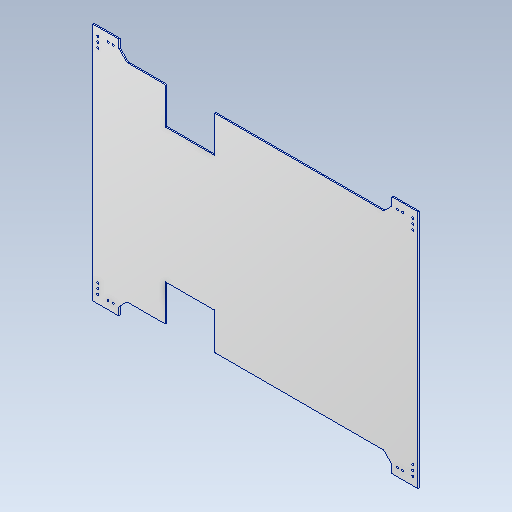
# Autodesk Inventor part: BELLYPAN
Saved by Autodesk Inventor 2020 (Build 240168000, 168)
## iProperties
Created: 2021-01-06
Part Number: BELLYPAN
Material: Aluminum 6061
Document SubType Name: Modeling
Designer: lucky
Density: 2.7 g/cm^3
Appearance: Aluminum - Flat
Mass: 3216.38 g
Surface Area: 8048.59 cm^2
Volume: 1191.25 cm^3
Author: lucky
Autodesk Inventor part; units mm, degrees
ref_plane "YZ Plane" through (0, 0, 0) normal (1, 0, 0) x (0, 1, 0)
ref_plane "XZ Plane" through (0, 0, 0) normal (0, 1, 0) x (-1, 0, 0)
ref_plane "XY Plane" through (0, 0, 0) normal (0, 0, 1) x (1, 0, 0)
sketch "Sketch1" plane through (0, 0, 0) normal (0, 0, 1) x (1, 0, 0)
  line L0 (775, 52) -> (25, 52) projected
  line L1 (0, 0) -> (0, 700) projected
  line L2 (0, 52) -> (800, 52)
  line L3 (800, 52) -> (800, 642)
  line L4 (800, 642) -> (0, 642)
  line L5 (0, 642) -> (0, 52)
  point P0 (0, 642)
  dimension "d0" = 800
  dimension "d1" = 590
  constraints: 8 end point, 2 parallel, 1 horizontal, 1 perpendicular, 1 point on line
  measures "d0" distance between parallel lines of L3 L1
  measures "d1" distance between parallel lines of L0 L4
extrude "Extrusion1" add sketch "Sketch1" along normal blind 3
sketch "Sketch2" plane through (0, 0, 3) normal (0, 0, 1) x (1, 0, 0)
  line L0 (25, 642) -> (775, 642) projected
  line L1 (671.5125, 642) -> (700.0875, 642) projected
  line L2 (800, 642) -> (0, 642) projected
  line L3 (735.75, 642) -> (64.25, 642)
  line L4 (64.25, 642) -> (64.25, 622)
  line L5 (84.25, 602) -> (715.75, 602)
  line L6 (735.75, 622) -> (735.75, 642)
  line L7 (800, 52) -> (800, 642) projected
  line L8 (0, 642) -> (0, 52) projected
  line L9 (0, 52) -> (800, 52) projected
  line L10 (735.75, 52) -> (64.25, 52)
  line L11 (64.25, 52) -> (64.25, 72)
  line L12 (84.25, 92) -> (715.75, 92)
  line L13 (735.75, 72) -> (735.75, 52)
  line L14 (25, 602) -> (775, 602) projected
  line L15 (270.7648, 597) -> (270.7648, 602) projected
  line L16 (178.8488, 568.7508) -> (178.8488, 563.7508) projected
  line L17 (178.2661, 125.2492) -> (178.2661, 130.2492) projected
  line L18 (299.9157, 125.2492) -> (299.9157, 130.2492) projected
  line L19 (300.4983, 568.7508) -> (300.4983, 563.7508) projected
  line L20 (298.8488, 602) -> (178.8488, 602)
  line L21 (178.8488, 602) -> (178.8488, 512)
  line L22 (178.8488, 512) -> (298.8488, 512)
  line L23 (298.8488, 512) -> (298.8488, 602)
  line L24 (800, 347) -> (0, 347) construction
  line L25 (178.8488, 92) -> (178.8488, 182)
  line L26 (178.8488, 182) -> (298.8488, 182)
  line L27 (298.8488, 182) -> (298.8488, 92)
  line L28 (64.25, 622) -> (84.25, 602)
  line L29 (735.75, 622) -> (715.75, 602)
  line L30 (84.25, 92) -> (64.25, 72)
  line L31 (715.75, 92) -> (735.75, 72)
  point P0 (0, 0)
  point P1 (64.25, 602)
  point P2 (735.75, 602)
  point P3 (64.25, 92)
  point P4 (735.75, 92)
  point P5 (64.25, 632)
  point P6 (64.25, 62)
  point P7 (400, 602)
  point P8 (400, 642)
  point P9 (735.75, 642)
  point P10 (64.25, 642)
  point P11 (178.8488, 557)
  point P12 (178.8488, 566.2508)
  dimension "d4" = 40
  dimension "d5" = 510
  dimension "d7" = 671.5
  dimension "d10" = 90
  dimension "d11" = 120
  dimension "d19" = 20
  dimension "d20" = 20
  dimension "d21" = 20
  dimension "d22" = 20
  dimension "d23" = 20
  dimension "d24" = 20
  dimension "d25" = 20
  dimension "d26" = 20
  constraints: 40 end point, 11 point on line, 8 midpoint, 7 parallel, 4 symmetric about line, 3 horizontal, 3 perpendicular, 3 vertical alignment
  measures "d4" distance between parallel lines of L5 L0
  measures "d5" distance between parallel lines of L12 L5
  measures "d7" distance between parallel lines of L4 L6
  measures "d10" distance between parallel lines of L20 L22
  measures "d11" distance between parallel lines of L21 L23
  measures "d19" distance of L4.end point (64.25, 602)
  measures "d20" distance of L5.start point (64.25, 602)
  measures "d21" distance of L6.start point (735.75, 602)
  measures "d22" distance of L5.end point (735.75, 602)
  measures "d23" distance of L12.start point (64.25, 92)
  measures "d24" distance of L11.end point (64.25, 92)
  measures "d25" distance of L12.end point (735.75, 92)
  measures "d26" distance of L13.start point (735.75, 92)
extrude "Extrusion2" cut sketch "Sketch2" against normal blind 10 contours L0 L6 L29 L5 L28 L4 | L11 L30 L12 L31 L13 L9 | L5 L23 L22 L21 L16 | L25 L26 L27 L12
sketch "Sketch3" plane through (0, 0, 3) normal (0, 0, 1) x (1, 0, 0)
  circle A0 centre (12.5, 72) radius 2.5 projected
  circle A1 centre (37.5, 72) radius 2.5 projected
  circle A2 centre (50, 72) radius 2.5 projected
  circle A3 centre (12.5, 97) radius 2.5 projected
  circle A4 centre (12.5, 84.5) radius 2.5 projected
  line L0 (64.25, 622) -> (64.25, 642) projected
  line L1 (64.25, 642) -> (0, 642) projected
  line L2 (0, 642) -> (0, 52) projected
  line L3 (0, 52) -> (64.25, 52) projected
  line L4 (64.25, 52) -> (64.25, 72) projected
  line L5 (84.25, 92) -> (178.8488, 92) projected
  line L6 (178.8488, 92) -> (178.8488, 182) projected
  line L7 (178.8488, 182) -> (298.8488, 182) projected
  line L8 (298.8488, 182) -> (298.8488, 92) projected
  line L9 (298.8488, 92) -> (715.75, 92) projected
  line L10 (735.75, 72) -> (735.75, 52) projected
  line L11 (735.75, 52) -> (800, 52) projected
  line L12 (800, 52) -> (800, 642) projected
  line L13 (800, 642) -> (735.75, 642) projected
  line L14 (735.75, 642) -> (735.75, 622) projected
  line L15 (715.75, 602) -> (298.8488, 602) projected
  line L16 (298.8488, 602) -> (298.8488, 512) projected
  line L17 (298.8488, 512) -> (178.8488, 512) projected
  line L18 (178.8488, 512) -> (178.8488, 602) projected
  line L19 (178.8488, 602) -> (84.25, 602) projected
  circle A5 centre (12.5, 622) radius 2.5 projected
  circle A6 centre (37.5, 622) radius 2.5 projected
  circle A7 centre (50, 622) radius 2.5 projected
  circle A8 centre (12.5, 609.5) radius 2.5 projected
  circle A9 centre (12.5, 597) radius 2.5 projected
  circle A10 centre (750, 622) radius 2.5 projected
  circle A11 centre (762.5, 622) radius 2.5 projected
  circle A12 centre (787.5, 622) radius 2.5 projected
  circle A13 centre (787.5, 609.5) radius 2.5 projected
  circle A14 centre (787.5, 597) radius 2.5 projected
  circle A15 centre (750, 72) radius 2.5 projected
  circle A16 centre (762.5, 72) radius 2.5 projected
  circle A17 centre (787.5, 72) radius 2.5 projected
  circle A18 centre (787.5, 84.5) radius 2.5 projected
  circle A19 centre (787.5, 97) radius 2.5 projected
  line L20 (64.25, 72) -> (84.25, 92) projected
  line L21 (715.75, 92) -> (735.75, 72) projected
  line L22 (735.75, 622) -> (715.75, 602) projected
  line L23 (84.25, 602) -> (64.25, 622) projected
  point P0 (0, 0)
hole "Hole1" at (50, 72, 3) at (37.5, 72, 3) at (12.5, 72, 3) at (12.5, 84.5, 3) at (12.5, 97, 3) at (12.5, 597, 3) at (12.5, 609.5, 3) at (12.5, 622, 3) at (37.5, 622, 3) at (50, 622, 3) at (750, 622, 3) at (762.5, 622, 3) at (787.5, 622, 3) at (787.5, 609.5, 3) at (787.5, 597, 3) at (750, 72, 3) at (762.5, 72, 3) at (787.5, 72, 3) at (787.5, 84.5, 3) at (787.5, 97, 3) direction (0, 0, -1) diameter 5 depth 10
fillet "Fillet1" radius 2 4 edges at (178.8488, 602, 1.5) (298.8488, 602, 1.5) (178.8488, 92, 1.5) (298.8488, 92, 1.5)
equation "\"d0\" = Chassi_Length"
equation "\"d1\" = Chassi_Width - 2 * WheelBay_Depth"
equation "\"d4\" = RHS_Width"
equation "\"d5\" = -2 * WheelBay_Depth + Chassi_Width - 2 * RHS_Width"
equation "\"d20\" = d19"
equation "\"d21\" = d19"
equation "\"d22\" = d21"
equation "\"d23\" = d19"
equation "\"d24\" = d23"
equation "\"d25\" = d19"
equation "\"d26\" = d25"
equation "\"Chassi_Length\" = 800"
equation "\"Chassi_CentreDrop\" = 4"
equation "\"WheelBay_Depth\" = 55"
equation "\"Wheel_Diametre\" = 152.4"
equation "\"Wheel_Seperation\" = 285.75"
equation "\"Wheel_HeightOffset\" = 4"
equation "\"Wheel_Clearance\" = 13.05"
equation "\"RHS_Width\" = 40"
equation "\"Chassi_GroundClearance\" = 10.116"
equation "\"Wheel_CentreDrop\" = 4"
equation "\"Wheel_Seperation2\" = 194.33333"
equation "\"Wheel_Diametre2\" = 101.6"
equation "\"Wheel_HeightOffset2\" = 4"
equation "\"Wheel_Clearance2\" = 32.7"
equation "\"Chain_Pitch\" = 9.525"
equation "\"Wheel_MaxSeperation\" = 285.75"
equation "\"Wheel_CCSpan\" = 571.5"
equation "\"Wheel_CCSpan2\" = 471.5"
equation "\"Wheel_MaxSeperation2\" = 190.5"
equation "\"MotorholeCC\" = 95.25"
equation "\"MotorholeHorizontal\" = 95.01318"
equation "\"OutputshaftTopOffset\" = 30.058"
equation "\"Heightfromcenter\" = 6.7125"
equation "\"Chassi_SideRivetSpacing\" = 37.5"
equation "\"Sprocket_Thickness\" = 10.668"
equation "\"BumperMountingBarOffset\" = 177.8"
equation "\"Chassi_Width\" = 700"
body "Solid1"
